herzal_v2 (Autodesk Fusion 360 design; units mm, degrees)
Autodesk Fusion 360 part; units mm, degrees
note: some values were not read from the file. Chosen so that the rebuilt part matches the saved one: which face or edge a step refers to. Set by a fixed rule: which sketch regions a step uses.
sketch "Sketch1" plane through (0, 0, 0) normal (0, 1, 0) x (1, 0, 0)
  circle A0 centre (0, 0) radius 5.5
  circle A1 centre (-11, 0) radius 5.5
  line L0 (0, 5.5) -> (0, -16.5)
  line L1 (0, -16.5) -> (-15, -16.5)
  line L2 (-5.5, 0) -> (-5.5, -17)
  line L3 (-16.5, 0) -> (5.5, 0)
  line L4 (-5.5, -16.5) -> (-15.4, -3.3)
  line L5 (-5.5, -16.5) -> (4.4, -3.3)
  dimension "d1" = 11
  dimension "d2" = 11
  dimension "d3" = 22
  constraint coincident A0.centre origin
  constraint coincident A0 L0.start
  constraint vertical L0
  constraint perpendicular L0 L1
  constraint coincident A1 L2.start
  constraint coincident A0 L2.start
  constraint tangent A0 L2
  constraint perpendicular L1 L2
  constraint coincident A1 L3.start
  constraint coincident A0 L3.end
  constraint horizontal L3
  constraint coincident L1 L4.start
  constraint coincident L2 L4.start
  constraint coincident A1 L4.end
  constraint tangent A1 L4
  constraint coincident A0 L5.end
  constraint tangent A0 L5
  measures "d1" diameter of A0
  measures "d2" diameter of A1
  measures "d3" distance of L0.start L0.end
extrude "Extrude1" add sketch "Sketch1" along normal blind 20 contours A0 L0 L3 | A0 L0 L3 | A0 L0 L3 | A0 L0 L5 | A0 L0 L3 | A1 L3 | A1 L2 L4 | A0 L0 L2 L5 | A1 L3 makes body 1
fillet "Fillet1" radius 0.75 1 edges at (-5.5, 10, 0) on bodies 1
fillet "Fillet2" radius 0.5 1 edges at (-5.5, 10, 16.5) on bodies 1
copy_body "CopyPasteBodies3" bodies 1 makes body 2
scale "Scale2" factors (1.1, 1, 1.1) about (-6.16, 0, -2.6124) bodies 2
move_body "Move2" bodies 2 to x (1, 0, 0) y (0, 1, 0) z (0, 0, 1) at (0, 0, -0.8)
copy_body "CopyPasteBodies4" bodies 1 makes body 3
move_face "OffsetFaces1" offset 0.8 4 faces at (-9.0667, 13.3333, 11.7444) (-6.4441, 6.6667, -3.0811) (-1.9333, 13.3333, 11.7444) (-4.5559, 6.6667, -3.0811) on bodies 3
fillet "Fillet3" radius 1 1 edges at (-5.5, 10, -3.0725) on bodies 3
combine "Combine1" operation cut target body 3 tool bodies 1 keep tools result as body 4 in component "Component"
component "Component" placed x (1, 0, 0) y (0, 1, 0) z (0, 0, 1) at (0, 0, 0)
